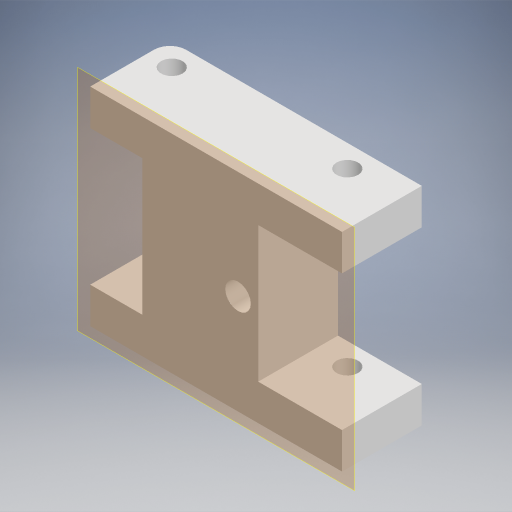
# Autodesk Inventor part: front ankle connection_left
Saved by Autodesk Inventor 2024 (Build 280153000, 153)
## iProperties
Created: 2024-09-16
Part Number: front ankle connection_left
Material: 일반
Document SubType Name: Modeling
Designer: msi
Density: 1 g/cm^3
Appearance: 기본값
Author: msi
Autodesk Inventor part; units mm, degrees
ref_plane "YZ Plane" through (0, 0, 0) normal (1, 0, 0) x (0, 1, 0)
ref_plane "XZ Plane" through (0, 0, 0) normal (0, 1, 0) x (-1, 0, 0)
ref_plane "XY Plane" through (0, 0, 0) normal (0, 0, 1) x (1, 0, 0)
ref_plane "작업 평면2" through (0, 0, 0) normal (0, 0, 1) x (1, 0, 0)
sketch "스케치2" plane through (0, 0, 0) normal (0, 0, 1) x (1, 0, 0)
  line L0 (-9.2237, -8.5) -> (-9.2237, 8.5) projected
  line L1 (-15.7763, -8.5) -> (-9.2237, -8.5) projected
  line L2 (-15.7763, -13) -> (-15.7763, -8.5) projected
  line L3 (15.7763, -13) -> (-15.7763, -13) projected
  line L4 (15.7763, -8.5) -> (15.7763, -13) projected
  line L5 (5.2737, -8.5) -> (15.7763, -8.5) projected
  line L6 (5.2737, 8.5) -> (5.2737, -8.5) projected
  line L7 (15.7763, 8.5) -> (5.2737, 8.5) projected
  line L8 (15.7763, 13) -> (15.7763, 8.5) projected
  line L9 (-15.7763, 13) -> (15.7763, 13) projected
  line L10 (-15.7763, 8.5) -> (-15.7763, 13) projected
  line L11 (-9.2237, 8.5) -> (-15.7763, 8.5) projected
  circle A0 centre (2.7487, -0.5) radius 1.6 projected
  line L12 (15.7763, 13) -> (-15.7763, 13)
  line L13 (-15.7763, 13) -> (-15.7763, 8.5)
  line L14 (-15.7763, 8.5) -> (15.7763, 8.5)
  line L15 (15.7763, 8.5) -> (15.7763, 13)
  line L16 (5.2737, 8.5) -> (-9.2237, 8.5)
  line L17 (-9.2237, 8.5) -> (-9.2237, -8.5)
  line L18 (-9.2237, -8.5) -> (5.2737, -8.5)
  line L19 (5.2737, -8.5) -> (5.2737, 8.5)
  line L20 (15.7763, -8.5) -> (-15.7763, -8.5)
  line L21 (-15.7763, -8.5) -> (-15.7763, -13)
  line L22 (-15.7763, -13) -> (15.7763, -13)
  line L23 (15.7763, -13) -> (15.7763, -8.5)
  point P0 (0, 0)
  constraints: 24 end point, 6 parallel, 3 horizontal, 3 perpendicular
extrude "돌출1" add sketch "스케치2" against normal blind 10
sketch "스케치3" plane through (-15.7763, 13, 0) normal (0, 1, 0) x (1, 0, 0)
  arc A0 (2, 10) -> (0, 8) centre (2, 8) ccw projected
  line L0 (0, 8) -> (0, 0) projected
  line L1 (0, 0) -> (31.5525, 0) projected
  line L2 (31.5525, 10) -> (31.5525, 0) projected
  line L3 (2, 10) -> (31.5525, 10) projected
  circle A1 centre (3.025, 7.2) radius 1.35 projected
  circle A2 centre (25.025, 7.2) radius 1.35 projected
  circle A3 centre (25.025, 7.2) radius 1.35
  circle A4 centre (3.025, 7.2) radius 1.35
  point P0 (15.7763, 0)
  constraints: 2 centre point, 2 coincident, 2 concentric
extrude "돌출2" cut sketch "스케치3" against normal through all contours A1 | A2
fillet "모깎기1" radius 2 2 edges at (-15.7763, -10.75, -10) (-15.7763, 10.75, -10)
